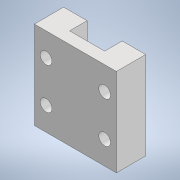
# Autodesk Inventor part: sub_arm_2
Saved by Autodesk Inventor 2020 (Build 240168000, 168)
## iProperties
Created: 2019-10-19
Part Number: sub_arm_2
Material: Generic
Document SubType Name: Modeling
Designer: psrob
Density: 1 g/cm^3
Appearance: Default
Author: psrob
Autodesk Inventor part; units mm, degrees
ref_plane "YZ Plane" through (0, 0, 0) normal (1, 0, 0) x (0, 1, 0)
ref_plane "XZ Plane" through (0, 0, 0) normal (0, 1, 0) x (-1, 0, 0)
ref_plane "XY Plane" through (0, 0, 0) normal (0, 0, 1) x (1, 0, 0)
sketch "Sketch1" plane through (0, 0, 0) normal (0, 0, 1) x (1, 0, 0)
  line L0 (7, 7.5) -> (3, 7.5) projected
  line L1 (3, 7.5) -> (3, -7.5) projected
  line L2 (7, -7.5) -> (3, -7.5) projected
  line L3 (7, 7.5) -> (7, -7.5) projected
  circle A0 centre (5, -3.5) radius 1 projected
  circle A1 centre (5, 3.5) radius 1 projected
  line L4 (-3, 7.5) -> (-7, 7.5) projected
  line L5 (-7, -7.5) -> (-7, 7.5) projected
  line L6 (-3, -7.5) -> (-7, -7.5) projected
  line L7 (-3, -7.5) -> (-3, 7.5) projected
  circle A2 centre (-5, 3.5) radius 1 projected
  circle A3 centre (-5, -3.5) radius 1 projected
  point P0 (0, 0)
extrude "Extrusion1" add sketch "Sketch1" along normal blind 3
sketch "Sketch2" plane through (0, 0, 3) normal (0, 0, 1) x (1, 0, 0)
  line L0 (7, -7.5) -> (7, 7.5) projected
  line L1 (7, 7.5) -> (3, 7.5) projected
  line L2 (3, 7.5) -> (3, -7.5) projected
  line L3 (3, -7.5) -> (7, -7.5) projected
  circle A0 centre (5, -3.5) radius 1 projected
  circle A1 centre (5, 3.5) radius 1 projected
  line L4 (-3, -7.5) -> (-3, 7.5) projected
  line L5 (-3, 7.5) -> (-7, 7.5) projected
  line L6 (-7, 7.5) -> (-7, -7.5) projected
  line L7 (-7, -7.5) -> (-3, -7.5) projected
  circle A2 centre (-5, 3.5) radius 1 projected
  circle A3 centre (-5, -3.5) radius 1 projected
  line L8 (7, -7.5) -> (-7, -7.5)
  line L9 (-7, -7.5) -> (-7, 7.5)
  line L10 (-7, 7.5) -> (7, 7.5)
  line L11 (7, 7.5) -> (7, -7.5)
  point P0 (0, 0)
  constraints: 8 end point, 2 parallel, 1 horizontal, 1 perpendicular
extrude "Extrusion2" add sketch "Sketch2" along normal blind 2
body "Solid1"
